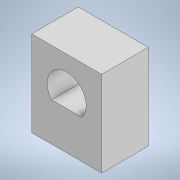
# Autodesk Inventor part: Hammer_Halter
Saved by Autodesk Inventor 2021 (Build 250183000, 183)
## iProperties
Created: 2024-05-15
Part Number: Hammer_Halter
Material: Generic
Document SubType Name: Modeling
Designer: Lukas
Density: 1 g/cm^3
Appearance: Default
Author: Lukas
Autodesk Inventor part; units mm, degrees
ref_plane "YZ Plane" through (0, 0, 0) normal (1, 0, 0) x (0, 1, 0)
ref_plane "XZ Plane" through (0, 0, 0) normal (0, 1, 0) x (-1, 0, 0)
ref_plane "XY Plane" through (0, 0, 0) normal (0, 0, 1) x (1, 0, 0)
sketch "Sketch1" plane through (0, 0, 0) normal (0, 0, 1) x (1, 0, 0)
  circle A0 centre (0, 0) radius 5
  line L0 (-9, 9) -> (9, 9)
  line L1 (9, 9) -> (9, -13)
  line L2 (9, -13) -> (-9, -13)
  line L3 (-9, -13) -> (-9, 9)
  line L4 (3.923, -3.1) -> (-3.923, -3.1)
  point P0 (0, 9)
  dimension "d1" = 10
  dimension "d2" = 18
  dimension "d3" = 9
  dimension "d4" = 13
  dimension "d18" = 3.1
  constraints: 10 end point, 2 horizontal, 2 parallel, 2 point on circle, 1 centre point, 1 coincident, 1 midpoint, 1 perpendicular, 1 vertical alignment
  measures "d1" diameter of A0
  measures "d2" distance of L0.start L0.end
  measures "d3" distance from line of point (0, 0) L0
  measures "d4" distance from line of L2 point (0, 0)
  measures "d18" distance from line of point (0, 0) L4
extrude "Extrusion1" add sketch "Sketch1" along normal blind 12 contours L4 A0 | L0 L1 L2 L3 picked at (-1.0435, -3.3662)
sketch "Sketch2" plane through (-9, -13, 0) normal (0, -1, 0) x (1, 0, 0)
  circle A0 centre (15, 6) radius 1.4
  circle A1 centre (3, 6) radius 1.4
  line L0 (18, 0) -> (18, 12) projected
  line L1 (0, 0) -> (0, 12) projected
  point P0 (9, 0)
  point P1 (18, 6)
  dimension "d7" = 2.8
  dimension "d8" = 3
  dimension "d9" = 3
  constraints: 2 centre point, 2 horizontal alignment, 1 equal radius, 1 midpoint
  measures "d7" diameter of A0
  measures "d8" distance from line of L0 A0.centre
  measures "d9" distance from line of L1 A1.centre
extrude "Extrusion2" cut sketch "Sketch2" against normal blind 8
equation "\"d3\" = 0.5 * d2"
equation "\"d9\" = d8"
body "Solid1"
